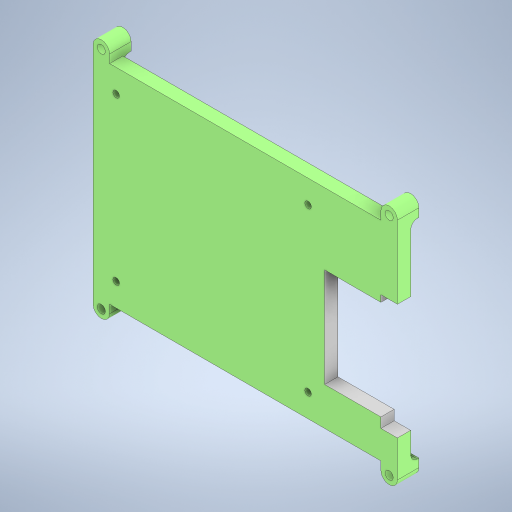
# Autodesk Inventor part: 라즈베리파이 고정 커버
Saved by Autodesk Inventor 2023.1 (Build 271208000, 208)
## iProperties
Created: 2022-08-09
Part Number: 라즈베리파이 고정 커버
Material: 일반
Document SubType Name: Modeling
Designer: fly01
Density: 1 g/cm^3
Appearance: 기본값
Author: fly01
Autodesk Inventor part; units mm, degrees
ref_plane "YZ Plane" through (0, 0, 0) normal (1, 0, 0) x (0, 1, 0)
ref_plane "XZ Plane" through (0, 0, 0) normal (0, 1, 0) x (-1, 0, 0)
ref_plane "XY Plane" through (0, 0, 0) normal (0, 0, 1) x (1, 0, 0)
sketch "스케치1" plane through (0, 0, 0) normal (0, 0, 1) x (1, 0, 0)
  line L0 (-46, -31.5) -> (46, -31.5)
  line L1 (46, -31.5) -> (46, 31.5)
  line L2 (46, 31.5) -> (-46, 31.5)
  line L3 (-46, 31.5) -> (-46, -31.5)
  line L4 (-46, -31.5) -> (46, 31.5) construction
  line L5 (46, -31.5) -> (-46, 31.5) construction
  line L6 (-42.5, 28) -> (42.5, 28) construction
  line L7 (42.5, 28) -> (42.5, -28) construction
  line L8 (42.5, -28) -> (-42.5, -28) construction
  line L9 (-42.5, -28) -> (-42.5, 28) construction
  line L10 (-42.5, 28) -> (42.5, -28) construction
  line L11 (42.5, 28) -> (-42.5, -28) construction
  circle A0 centre (-39, -24.5) radius 1
  circle A1 centre (19, -24.5) radius 1
  line L12 (0, 0) -> (14.8173, 0)
  circle A2 centre (-39, 24.5) radius 1
  circle A3 centre (19, 24.5) radius 1
  line L13 (-46, 31.5) -> (-41, 31.5)
  line L14 (-41, 31.5) -> (-41, 34)
  line L15 (-41, 34) -> (-46, 34) construction
  line L16 (-46, 34) -> (-46, 31.5)
  circle A4 centre (-43.5, 34) radius 2.5
  circle A5 centre (-43.5, 34) radius 1.25
  line L17 (0, 0) -> (0, 10.4922)
  line L18 (46, 31.5) -> (41, 31.5)
  line L19 (41, 31.5) -> (41, 34)
  line L20 (41, 34) -> (46, 34) construction
  line L21 (46, 34) -> (46, 31.5)
  circle A6 centre (43.5, 34) radius 2.5
  circle A7 centre (43.5, 34) radius 1.25
  line L22 (46, -31.5) -> (-46, -31.5)
  line L23 (-46, -31.5) -> (-41, -31.5)
  line L24 (-41, -31.5) -> (-41, -34)
  line L25 (-41, -34) -> (-46, -34) construction
  line L26 (-46, -34) -> (-46, -31.5)
  circle A8 centre (-43.5, -34) radius 2.5
  circle A9 centre (-43.5, -34) radius 1.25
  line L27 (41, -31.5) -> (41, -34)
  circle A10 centre (43.5, -34) radius 1.25
  line L28 (41, -34) -> (46, -34) construction
  line L29 (46, -34) -> (46, -31.5)
  circle A11 centre (43.5, -34) radius 2.5
  line L30 (46, -31.5) -> (41, -31.5)
  dimension "d0" = 92
  dimension "d1" = 63
  dimension "d2" = 85
  dimension "d3" = 56
  dimension "d4" = 3.5
  dimension "d5" = 3.5
  dimension "d6" = 2
  dimension "d7" = 2
  dimension "d8" = 58
  dimension "d9" = 3.5
  dimension "d10" = 5
  dimension "d11" = 2.5
  dimension "d12" = 2.5
  constraints: 62 end point, 17 symmetric about line, 8 centre point, 6 horizontal, 6 parallel, 5 midpoint, 4 coincident, 4 perpendicular, 1 vertical, 17 other
  measures "d0" distance of L2.end L1.end
  measures "d1" distance of L1.end L0.end
  measures "d2" distance of L7.end L8.end
  measures "d3" distance of L6.end L7.end
  measures "d4" distance from line of L9 A0.centre
  measures "d5" distance from line of L8 A0.centre
  measures "d6" diameter of A0
  measures "d7" diameter of A1
  measures "d8" distance of A0.centre A1.centre
  measures "d9" distance from line of L8 A1.centre
  measures "d10" distance of L14.end L15.end
  measures "d11" distance of L13.end L14.end
  measures "d12" diameter of A5
extrude "돌출1" add sketch "스케치1" along normal blind 4
sketch "스케치3" plane through (0, 0, 0) normal (0, 0, -1) x (-1, 0, 0)
  circle A0 centre (-19, 24.5) radius 1 projected
  circle A1 centre (-19, 24.5) radius 3
  circle A2 centre (39, 24.5) radius 1 projected
  circle A3 centre (39, 24.5) radius 3
  circle A4 centre (-19, -24.5) radius 1 projected
  circle A5 centre (-19, -24.5) radius 3
  circle A6 centre (39, -24.5) radius 1 projected
  circle A7 centre (39, -24.5) radius 3
  point P0 (0, 0)
  dimension "d24" = 6
  dimension "d25" = 6
  dimension "d26" = 6
  dimension "d27" = 6
  constraints: 4 centre point, 4 coincident
  measures "d24" diameter of A1
  measures "d25" diameter of A3
  measures "d26" diameter of A5
  measures "d27" diameter of A7
extrude "돌출3" add sketch "스케치3" along normal blind 2.5
extrude "돌출4" add sketch "스케치1" against normal blind 2.5 contours L24 A8 L0 | L0 A11 L27 | A8 L26 L0 | A8 | L0 L29 A11 | A11 | L16 A4 L2 | L2 A6 L21 | A4 L14 L2 | A4 | L2 L19 A6 | A6
fillet "모깎기1" radius 2 4 edges at (43.5, 31.5, 0) (-43.5, 31.5, 0) (43.5, -31.5, 0) (-43.5, -31.5, 0)
fillet "모깎기2" radius 1 4 edges at (22, 24.5, 0) (22, -24.5, 0) (-36, 24.5, 0) (-36, -24.5, 0)
sketch "스케치4" plane through (0, 0, 4) normal (0, 0, 1) x (1, 0, 0)
  line L0 (-46, 34) -> (-46, -34) projected
  line L1 (46, -29.5) -> (46, 29.5) projected
  line L2 (46, -34) -> (46, 34) projected
  line L3 (46, -20) -> (24, -20)
  line L4 (24, -20) -> (24, 10)
  line L5 (24, 10) -> (46, 10)
  line L6 (46, 10) -> (46, -20)
  line L7 (46, -20) -> (41, -20)
  line L8 (41, -20) -> (41, -23)
  line L9 (41, -23) -> (46, -23)
  line L10 (46, -23) -> (46, -20)
  line L11 (46, 10) -> (41, 10)
  line L12 (41, 10) -> (41, 12)
  line L13 (41, 12) -> (46, 12)
  line L14 (46, 12) -> (46, 10)
  point P0 (46, 0)
  point P1 (46, -20)
  point P2 (46, 10)
  point P3 (46, 0)
  dimension "d40" = 30
  dimension "d42" = 10
  dimension "d43" = 3
  dimension "d44" = 5
  dimension "d45" = 22
  dimension "d46" = 5
  dimension "d47" = 2
  constraints: 24 end point, 6 parallel, 3 horizontal, 3 perpendicular, 2 midpoint, 1 point on line
  measures "d40" distance of L3.end L4.end
  measures "d42" distance from line of point (46, 0) L5
  measures "d43" distance between parallel lines of L3 L9
  measures "d44" distance of L8.end L9.end
  measures "d45" distance of L4.end L5.end
  measures "d46" distance of L12.end L13.end
  measures "d47" distance of L11.end L12.end
extrude "돌출5" cut sketch "스케치4" against normal blind 10
